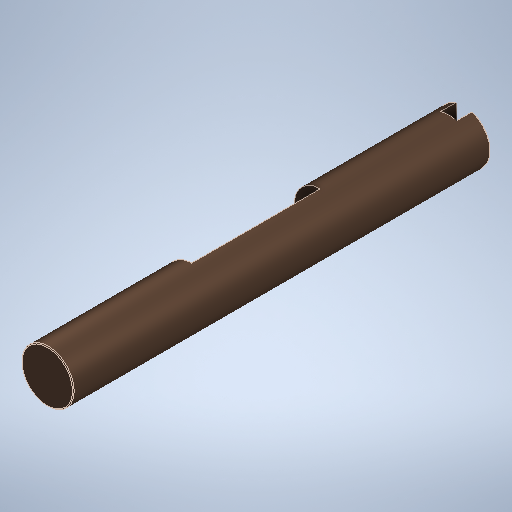
# Autodesk Inventor part: 26A - Valve
Saved by Autodesk Inventor 2025.2 (Build 292293000, 293)
## iProperties
Created: 2025-07-17
Part Number: 26A - Valve
Material: Bronze, Soft Tin
Document SubType Name: Modeling
Designer: bless
Density: 8.874 g/cm^3
Appearance: Bronze - Satin
Author: bless
Autodesk Inventor part; units mm, degrees
ref_plane "YZ Plane" through (0, 0, 0) normal (1, 0, 0) x (0, 1, 0)
ref_plane "XZ Plane" through (0, 0, 0) normal (0, 1, 0) x (-1, 0, 0)
ref_plane "XY Plane" through (0, 0, 0) normal (0, 0, 1) x (1, 0, 0)
sketch "Sketch1" plane through (0, 0, 0) normal (0, 0, 1) x (1, 0, 0)
  circle A0 centre (0, 0) radius 3.25
  dimension "d0" = 6.5
  constraints: 1 centre point, 1 coincident
  measures "d0" diameter of A0
extrude "Extrusion1" add sketch "Sketch1" against normal blind 18
sketch "Sketch2" plane through (0, 0, -18) normal (0, 0, -1) x (-1, 0, 0)
  circle A0 centre (0, 0) radius 3.25 projected
  circle A1 centre (0, 0) radius 3.25 projected
  line L0 (0, -3.25) -> (0, 3.25)
  constraints: 2 end point, 2 point on circle, 1 midpoint, 1 vertical
extrude "Extrusion2" add sketch "Sketch2" along normal blind 16 contours L0 A0 picked at (-1.3347, 0.1621)
sketch "Sketch3" plane through (0, 0, -34) normal (0, 0, -1) x (-1, 0, 0)
  arc A0 (0, 3.25) -> (0, -3.25) centre (0, 0) ccw projected
  circle A1 centre (0, 0) radius 3.25
  point P0 (0, -3.25)
  constraints: 1 centre point, 1 coincident, 1 concentric
extrude "Extrusion3" add sketch "Sketch3" along normal blind 18
sketch "Sketch4" plane through (0, 0, -52) normal (0, 0, -1) x (-1, 0, 0)
  circle A0 centre (0, 0) radius 3.25 projected
  line L0 (1, 4.2353) -> (-1, 4.2353)
  line L1 (-1, 4.2353) -> (-1, -4.2353)
  line L2 (-1, -4.2353) -> (1, -4.2353)
  line L3 (1, -4.2353) -> (1, 4.2353)
  line L4 (1, 4.2353) -> (-1, -4.2353) construction
  line L5 (-1, 4.2353) -> (1, -4.2353) construction
  point P0 (1, -3.0923)
  point P1 (1, 3.0923)
  point P2 (-1, 3.0923)
  point P3 (-1, -3.0923)
  dimension "d7" = 2
  dimension "d8" = 13.285
  constraints: 12 end point, 2 midpoint, 2 parallel, 1 horizontal, 1 perpendicular
  measures "d7" distance between parallel lines of L1 L3
  measures "d8" angle of L4 L3
extrude "Extrusion4" cut sketch "Sketch4" against normal blind 2 contours L3 A0 L1
chamfer "Chamfer1" distance 0.1 angle 45 3 edges at (-3.25, 0, 0) (-3.25, 0, -52) (3.25, 0, -52)
body "Solid1"
